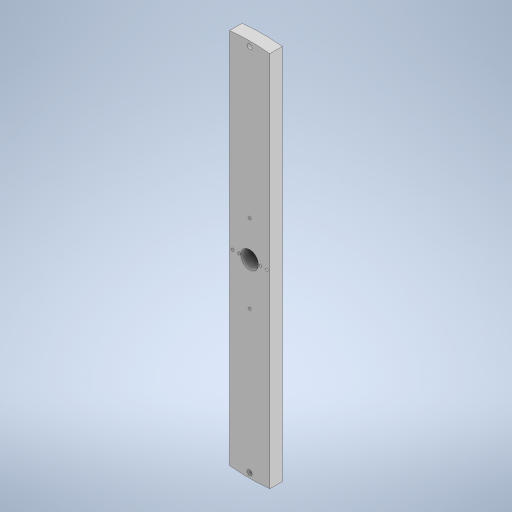
# Autodesk Inventor part: 상단 서보모터 고정 판
Saved by Autodesk Inventor 2023.1 (Build 271208000, 208)
## iProperties
Created: 2022-08-14
Part Number: 상단 서보모터 고정 판
Material: 일반
Document SubType Name: Modeling
Designer: fly01
Density: 1 g/cm^3
Appearance: 기본값
Author: fly01
Autodesk Inventor part; units mm, degrees
ref_plane "YZ Plane" through (0, 0, 0) normal (1, 0, 0) x (0, 1, 0)
ref_plane "XZ Plane" through (0, 0, 0) normal (0, 1, 0) x (-1, 0, 0)
ref_plane "XY Plane" through (0, 0, 0) normal (0, 0, 1) x (1, 0, 0)
sketch "스케치1" plane through (0, 0, 0) normal (0, 0, 1) x (1, 0, 0)
  line L0 (-8, -75.5) -> (8, -75.5)
  line L1 (8, -75.5) -> (8, 75.5)
  line L2 (8, 75.5) -> (-8, 75.5)
  line L3 (-8, 75.5) -> (-8, -75.5)
  line L4 (-8, -75.5) -> (8, 75.5) construction
  line L5 (8, -75.5) -> (-8, 75.5) construction
  circle A0 centre (0, 0) radius 75.5
  circle A1 centre (0, 73.5) radius 1
  line L6 (0, 0) -> (8, 0) construction
  circle A2 centre (0, -73.5) radius 1
  circle A3 centre (0, 0) radius 3.5
  circle A4 centre (-4.25, 0) radius 0.5
  circle A5 centre (-6.85, 0) radius 0.5
  line L7 (0, 0) -> (0, 3.196) construction
  circle A6 centre (4.25, 0) radius 0.5
  circle A7 centre (6.85, 0) radius 0.5
  circle A8 centre (0, 14.3) radius 0.5
  circle A9 centre (0, -16.9) radius 0.5
  point P0 (0, 75.5)
  point P1 (8, -75.075)
  point P2 (8, 75.075)
  point P3 (-8, 75.075)
  point P4 (-8, -75.075)
  dimension "d1" = 151
  dimension "d0" = 16
  dimension "d2" = 2
  dimension "d3" = 73.5
  dimension "d4" = 7
  dimension "d5" = 1
  dimension "d6" = 1
  dimension "d7" = 8.5
  dimension "d8" = 12.7
  dimension "d9" = 1
  dimension "d13" = 14.3
  dimension "d14" = 1
  dimension "d15" = 16.9
  constraints: 16 end point, 9 centre point, 4 midpoint, 3 symmetric about line, 2 coincident, 2 parallel, 1 horizontal, 1 perpendicular, 1 vertical, 6 other
  measures "d0" distance of L2.end L1.end
  measures "d2" diameter of A1
  measures "d3" distance of point (0, 0) A1.centre
  measures "d4" diameter of A3
  measures "d5" diameter of A4
  measures "d6" diameter of A5
  measures "d7" distance of A6.centre A4.centre
  measures "d9" diameter of A8
  measures "d13" distance of point (0, 0) A8.centre
  measures "d14" diameter of A9
  measures "d15" distance of A9.centre point (0, 0)
extrude "돌출1" add sketch "스케치1" along normal blind 5 contours A0 L3 L1
